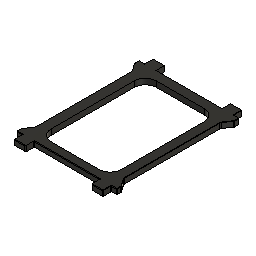
Rama fata-spate (Autodesk Fusion 360 design; units mm, degrees)
part number: 2026-05-26-13-04-27-356
Autodesk Fusion 360 part; units mm, degrees
sketch "Sketch1" plane through (0, 0, 0) normal (0, 0, 1) x (1, 0, 0)
  line L0 (-23, 48.647989) -> (-57, 48.647989)
  line L1 (-65, 56.647989) -> (-65, 115.647989)
  line L2 (-15, 56.647989) -> (-15, 115.647989)
  line L3 (-23, 123.647989) -> (-57, 123.647989)
  arc A0 (-65, 56.647989) -> (-57, 48.647989) centre (-57, 56.647989) ccw
  arc A1 (-57, 123.647989) -> (-65, 115.647989) centre (-57, 115.647989) ccw
  arc A2 (-23, 48.647989) -> (-15, 56.647989) centre (-23, 56.647989) ccw
  arc A3 (-15, 115.647989) -> (-23, 123.647989) centre (-23, 115.647989) ccw
  line L4 (-16.7, 43.000001) -> (-16.7, 37.000001)
  line L5 (-16.7, 37.000001) -> (-8.7, 37.000001)
  line L6 (-8.7, 37.000001) -> (-8.7, 43.000001)
  line L7 (-8.7, 43.000001) -> (-4.7, 43.000001)
  line L8 (-4.7, 43.000001) -> (-4.7, 45.984132)
  line L9 (-16.7, 43.000001) -> (-63.7, 43.000001)
  line L10 (-63.7, 43.000001) -> (-63.7, 37.000001)
  line L11 (-63.7, 37.000001) -> (-71.7, 37.000001)
  line L12 (-71.7, 37.000001) -> (-71.7, 43.000001)
  line L13 (-71.7, 43.000001) -> (-75.7, 43.000001)
  line L14 (-75.7, 43.000001) -> (-75.7, 45.984132)
  line L15 (-8.7, 52.631739) -> (-8.7, 120.368262)
  line L16 (-4.7, 127.01587) -> (-4.7, 130.000001)
  line L17 (-4.7, 130.000001) -> (-8.7, 130.000001)
  line L18 (-8.7, 130.000001) -> (-8.7, 136.000001)
  line L19 (-8.7, 136.000001) -> (-16.7, 136.000001)
  line L20 (-16.7, 136.000001) -> (-16.7, 130.000001)
  line L21 (-71.7, 52.631739) -> (-71.7, 120.368263)
  line L22 (-75.7, 127.01587) -> (-75.7, 130.000001)
  line L23 (-75.7, 130.000001) -> (-71.7, 130.000001)
  line L24 (-71.7, 130.000001) -> (-71.7, 136.000001)
  line L25 (-71.7, 136.000001) -> (-63.7, 136.000001)
  line L26 (-63.7, 136.000001) -> (-63.7, 130.000002)
  line L27 (-63.7, 130.000002) -> (-16.7, 130.000001)
  line L28 (-75.518557, 46.558557) -> (-72.062887, 51.482887)
  line L29 (-75.518557, 126.441444) -> (-72.062887, 121.517114)
  line L30 (-4.881443, 126.441444) -> (-8.337113, 121.517114)
  line L31 (-4.881443, 46.558557) -> (-8.337113, 51.482887)
  arc A4 (-75.518557, 46.558557) -> (-75.7, 45.984132) centre (-74.7, 45.984132) ccw
  arc A5 (-72.062887, 51.482887) -> (-71.7, 52.631739) centre (-73.7, 52.631739) ccw
  arc A6 (-71.7, 120.368263) -> (-72.062887, 121.517114) centre (-73.7, 120.368263) ccw
  arc A7 (-75.7, 127.01587) -> (-75.518557, 126.441444) centre (-74.7, 127.01587) ccw
  arc A8 (-4.881443, 126.441444) -> (-4.7, 127.01587) centre (-5.7, 127.01587) ccw
  arc A9 (-8.337113, 121.517114) -> (-8.7, 120.368262) centre (-6.7, 120.368262) ccw
  arc A10 (-4.7, 45.984132) -> (-4.881443, 46.558557) centre (-5.7, 45.984132) ccw
  arc A11 (-8.7, 52.631739) -> (-8.337113, 51.482887) centre (-6.7, 52.631739) ccw
  point P0 (-15, 48.647989)
  point P1 (-65, 48.647989)
  point P2 (-65, 123.647989)
  point P3 (-8.7, 52.000001)
  point P4 (-71.7, 52.000001)
  point P5 (-8.7, 121.000001)
  point P6 (-71.7, 121.000001)
  dimension "d1" = 50
  dimension "d2" = 75
  dimension "d3" = 8
  dimension "d4" = 8
  dimension "d5" = 8
  dimension "d6" = 8
  dimension "d8" = 8
  dimension "d9" = 6
  dimension "d10" = 4
  dimension "d20" = 47
  dimension "d21" = 6
  dimension "d22" = 8
  dimension "d23" = 6
  dimension "d24" = 4
  dimension "d28" = 69
  dimension "d31" = 4
  dimension "d32" = 6
  dimension "d33" = 8
  dimension "d34" = 6
  dimension "d35" = 69
  dimension "d38" = 4
  dimension "d39" = 6
  dimension "d40" = 8
  dimension "d45" = 1
  dimension "d46" = 2
  dimension "d47" = 2
  dimension "d48" = 1
  dimension "d49" = 1
  dimension "d50" = 2
  dimension "d51" = 1
  dimension "d52" = 2
  constraint horizontal L0
  constraint perpendicular L0 L1
  constraint perpendicular L0 L2
  constraint perpendicular L1 L3
  constraint tangent L1 A0
  constraint tangent L0 A0
  constraint tangent L1 A1
  constraint tangent L3 A1
  constraint tangent L0 A2
  constraint tangent L2 A2
  constraint tangent L3 A3
  constraint tangent L2 A3
  constraint perpendicular L4 L5
  constraint perpendicular L5 L6
  constraint perpendicular L6 L7
  constraint perpendicular L7 L8
  constraint perpendicular L4 L9
  constraint perpendicular L9 L10
  constraint perpendicular L10 L11
  constraint perpendicular L11 L12
  constraint perpendicular L12 L13
  constraint perpendicular L13 L14
  constraint perpendicular L16 L17
  constraint perpendicular L17 L18
  constraint perpendicular L18 L19
  constraint perpendicular L19 L20
  constraint perpendicular L22 L23
  constraint perpendicular L23 L24
  constraint perpendicular L24 L25
  constraint perpendicular L25 L26
  constraint tangent L14 A4
  constraint tangent L28 A4
  constraint tangent L28 A5
  constraint tangent L21 A5
  constraint tangent L21 A6
  constraint tangent L29 A6
  constraint tangent L29 A7
  constraint tangent L22 A7
  constraint tangent L30 A8
  constraint tangent L16 A8
  constraint tangent L15 A9
  constraint tangent L30 A9
  constraint tangent L8 A10
  constraint tangent L31 A10
  constraint tangent L31 A11
  constraint tangent L15 A11
  measures "d3" radius of A0
  measures "d4" radius of A1
  measures "d5" radius of A2
  measures "d6" radius of A3
  measures "d45" radius of A4
  measures "d46" radius of A5
  measures "d47" radius of A6
  measures "d48" radius of A7
  measures "d49" radius of A8
  measures "d50" radius of A9
  measures "d51" radius of A10
  measures "d52" radius of A11
extrude "Extrude1" add sketch "Sketch1" along normal blind 4 contours L4 L5 L6 L7 L8 L9 L10 L11 L12 L13 L14 L15 L16 L17 L18 L19 L20 L21 L22 L23 L24 L25 L26 L27 L28 L29 L30 L31 A4 A5 A6 A7 A8 A9 A10 A11 picked at (-69.466667, 96.215997)
chamfer "Chamfer1" distance 0.4 angle 45 5 faces at (-66.366667, 37.000001, 1.333333) (-14.033333, 37.000001, 1.333333) (-73.033333, 43.000001, 1.333333) (-32.366667, 43.000001, 1.333333) (-7.366667, 43.000001, 1.333333)
chamfer "Chamfer2" distance 0.2 angle 45 11 faces at (-8.7, 39.133334, 1.6) (-8.7, 75.21058, 1.333333) (-8.673433, 120.693164, 2.666667) (-6.033333, 124.800001, 1.333333) (-4.700832, 126.975087, 2.666667) (-4.7, 128.01058, 1.333333) (-8.594439, 51.990567, 2.666667) (-6.033333, 48.200001, 1.333333) (-4.799001, 46.417952, 2.666667) (-4.7, 44.261378, 1.333333) (-8.7, 132.000001, 1.333333)
chamfer "Chamfer3" distance 0.1 angle 45 5 faces at (-6.1, 130.000001, 1.466667) (-48.033333, 130.000001, 1.333333) (-11.5, 136.000001, 1.333333) (-69.033333, 136.000001, 1.333333) (-74.366667, 130.000001, 1.333333)
